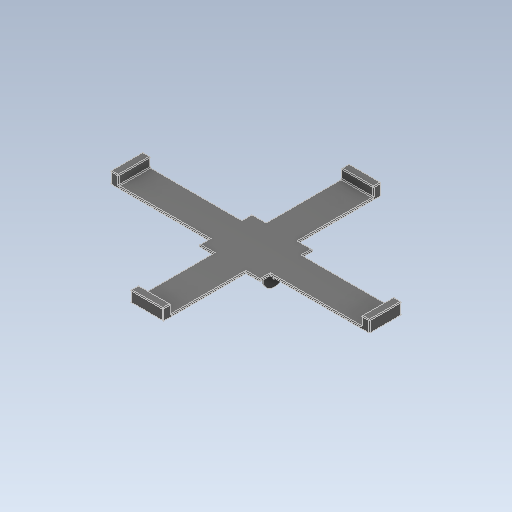
# Autodesk Inventor part: atassolar
Saved by Autodesk Inventor 2025.1 (Build 291241000, 241)
## iProperties
Created: 2024-11-08
Part Number: atassolar
Material: Aluminum 6061
Document SubType Name: Modeling
Designer: ramad
Density: 2.7 g/cm^3
Appearance: Aluminum - Flat
Author: ramad
Autodesk Inventor part; units mm, degrees
ref_plane "YZ Plane" through (0, 0, 0) normal (1, 0, 0) x (0, 1, 0)
ref_plane "XZ Plane" through (0, 0, 0) normal (0, 1, 0) x (-1, 0, 0)
ref_plane "XY Plane" through (0, 0, 0) normal (0, 0, 1) x (1, 0, 0)
sketch "Sketch1" plane through (0, 0, 0) normal (0, 1, 0) x (-1, 0, 0)
  line L0 (-43, 27.5) -> (43, 27.5)
  line L1 (43, 27.5) -> (43, -27.5)
  line L2 (43, -27.5) -> (-43, -27.5)
  line L3 (-43, -27.5) -> (-43, 27.5)
  line L4 (-43, 27.5) -> (43, -27.5) construction
  line L5 (43, 27.5) -> (-43, -27.5) construction
  line L6 (43, -27.5) -> (46, -27.5)
  line L7 (46, -27.5) -> (46, 27.5)
  line L8 (46, 27.5) -> (43, 27.5)
  line L9 (43, 27.5) -> (43, -27.5)
  line L10 (-43, -27.5) -> (-46, -27.5)
  line L11 (-46, -27.5) -> (-46, 27.5)
  line L12 (-46, 27.5) -> (-43, 27.5)
  line L13 (-43, 27.5) -> (-43, -27.5)
  point P0 (0, 0)
  dimension "d0" = 86
  dimension "d1" = 55
  dimension "d2" = 3
  dimension "d3" = 55
  dimension "d4" = 3
  constraints: 28 end point, 6 parallel, 3 horizontal, 3 perpendicular, 2 midpoint, 1 point on line
  measures "d0" distance of L1.end L2.end
  measures "d1" distance of L0.end L1.end
  measures "d2" distance of L8.end L7.end
  measures "d3" distance of L7.end L6.end
  measures "d4" distance of L11.end L12.end
extrude "Extrusion1" add sketch "Sketch1" along normal blind 3 contours L0 L1 L2 L3
extrude "Extrusion2" add sketch "Sketch1" along normal blind 3 contours L3 L10 L11 L12 | L8 L7 L6 L1
extrude "Extrusion3" add sketch "Sketch1" against normal blind 35 contours L3 L10 L11 L12 | L8 L7 L6 L1
sketch "Sketch2" plane through (46, 3, 27.5) normal (1, 0, 0) x (0, 0, -1)
  line L0 (0, -3) -> (0, -38) projected
  line L1 (0, -38) -> (55, -38) projected
  arc A0 (0, -38) -> (55, -38) centre (27.5, -28.794) ccw
  point P0 (27.5, -3)
  dimension "d11" = 29
  constraints: 2 point on circle, 1 centre point
  measures "d11" radius of A0
extrude "Extrusion4" add sketch "Sketch2" against normal up to surface (3 mm away)
mirror "Mirror1" about plane through (0, 0, 0) normal (1, 0, 0) of "Extrusion4"
sketch "Sketch3" plane through (-46, 3, -27.5) normal (-1, 0, 0) x (0, 0, 1)
  circle A0 centre (27.5, -38) radius 4.5
  point P0 (27.5, -3)
  point P1 (0, -38)
  dimension "d14" = 9
  constraints: 1 centre point, 1 horizontal alignment
  measures "d14" diameter of A0
extrude "Extrusion5" cut sketch "Sketch3" against normal blind 106.25
sketch "Sketch4" plane through (0, 3, 0) normal (0, 1, 0) x (1, 0, 0)
  line L0 (300, -250) -> (-300, -250)
  line L1 (-300, -250) -> (-300, 250)
  line L2 (-300, 250) -> (300, 250)
  line L3 (300, 250) -> (300, -250)
  line L4 (300, -250) -> (-300, 250) construction
  line L5 (-300, -250) -> (300, 250) construction
  line L6 (75, -65) -> (-75, -65)
  line L7 (-75, -65) -> (-75, 65)
  line L8 (-75, 65) -> (75, 65)
  line L9 (75, 65) -> (75, -65)
  line L10 (75, -65) -> (-75, 65) construction
  line L11 (-75, -65) -> (75, 65) construction
  line L12 (0, 250) -> (-40, 250)
  line L13 (-40, 250) -> (-40, 65)
  line L14 (0, 250) -> (40, 250)
  line L15 (40, 250) -> (40, 65)
  line L16 (300, 0) -> (300, 40)
  line L17 (300, 40) -> (75, 40)
  line L18 (300, 0) -> (300, -40)
  line L19 (300, -40) -> (75, -40)
  line L20 (0, -250) -> (-40, -250)
  line L21 (-40, -250) -> (-40, -65)
  line L22 (0, -250) -> (40, -250)
  line L23 (40, -250) -> (40, -65)
  line L24 (-300, 0) -> (-300, -40)
  line L25 (-300, -40) -> (-75, -40)
  line L26 (-300, 0) -> (-300, 40)
  line L27 (-300, 40) -> (-75, 40)
  line L28 (300, 40) -> (320, 40)
  line L29 (320, 40) -> (320, -40)
  line L30 (320, -40) -> (300, -40)
  line L31 (-300, 40) -> (-320, 40)
  line L32 (-320, 40) -> (-320, -40)
  line L33 (-320, -40) -> (-300, -40)
  line L34 (-40, 250) -> (-40, 270)
  line L35 (-40, 270) -> (40, 270)
  line L36 (40, 270) -> (40, 250)
  line L37 (-40, -250) -> (-40, -270)
  line L38 (-40, -270) -> (40, -270)
  line L39 (40, -270) -> (40, -250)
  point P0 (0, 0)
  dimension "d17" = 600
  dimension "d18" = 500
  dimension "d19" = 150
  dimension "d20" = 130
  dimension "d21" = 40
  dimension "d22" = 40
  dimension "d23" = 40
  dimension "d24" = 40
  dimension "d25" = 40
  dimension "d26" = 40
  dimension "d27" = 40
  dimension "d28" = 20
  dimension "d29" = 20
  dimension "d30" = 20
  dimension "d31" = 20
  constraints: 80 end point, 24 point on line, 13 perpendicular, 8 midpoint, 4 horizontal, 4 parallel
  measures "d17" distance of L1.end L2.end
  measures "d18" distance of L0.end L1.end
  measures "d19" distance of L7.end L8.end
  measures "d20" distance of L6.end L7.end
  measures "d21" distance of L12.start L12.end
  measures "d22" distance of L12.start L14.end
  measures "d23" distance of L16.start L16.end
  measures "d24" distance of L16.start L18.end
  measures "d25" distance of L20.start L20.end
  measures "d26" distance of L20.start L22.end
  measures "d27" distance of L24.start L24.end
  measures "d28" distance of L16.end L28.end
  measures "d29" distance of L26.end L31.end
  measures "d30" distance of L12.end L34.end
  measures "d31" distance of L20.end L37.end
extrude "Extrusion6" add sketch "Sketch4" along normal blind 5 contours L0 L21 L6 L23 | L19 L9 L17 L3 | L6 L7 L8 L9 | L1 L27 L7 L25 | L15 L8 L13 L2
extrude "Extrusion7" add sketch "Sketch4" along normal blind 28 contours L39 L38 L37 L0 | L3 L28 L29 L30 | L33 L32 L31 L1 | L2 L34 L35 L36
fillet "Fillet1" radius 2 53 edges at (-40, 8, -157.5) (-40, 19.5, -250) (40, 19.5, -250) (40, 8, -157.5) (-57.5, 8, -65) (-75, 8, -52.5) (-187.5, 8, -40) (-300, 19.5, -40) (-300, 19.5, 40) (-187.5, 8, 40) (-75, 8, 52.5) (-57.5, 8, 65) (-40, 8, 157.5) (187.5, 8, -40) (75, 8, -52.5) (57.5, 8, -65) (40, 8, 157.5) (57.5, 8, 65) (75, 8, 52.5) (187.5, 8, 40) (300, 19.5, 40) (300, 19.5, -40) (-40, 19.5, 250) (40, 19.5, 250) (-300, 31, 0) (0, 31, -250) (300, 31, 0) (0, 31, 250) (0, 31, 270) (-40, 31, 260) (-310, 31, 40) (-310, 31, -40) (40, 31, 260) (310, 31, 40) (310, 31, -40) (320, 31, 0) (-40, 31, -260) (40, 31, -260) (0, 31, -270) (-320, 31, 0) (-320, 17, 40) (-40, 17, -270) (40, 17, -270) (-320, 17, -40) (320, 17, -40) (320, 17, 40) (-40, 17, 270) (40, 17, 270) (0, 3, 270) (300, 8, 0) (0, 8, 250) (0, 8, -250) (-300, 8, 0)
body "Solid1"
